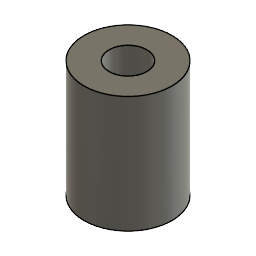
2tslot (Autodesk Fusion 360 archive; units mm, degrees)
design "nggonemotor"
part number: 2026-04-08-22-38-41-699
Autodesk Fusion 360 part; units mm, degrees
cylinder "CylinderPrimitive1" add diameter 18.6 height 24.7 placed x (1, 0, 0) y (0, 0, -1) z (0, 1, 0) at (0, 0, 0)
hole "Hole1" at (0, 24.7, 0) direction (0, -1, 0) diameter 8 depth 10 tip angle 180
hole "Hole2" at (0, 0, 0) direction (0, 1, 0) diameter 4.7 depth 10 tip angle 180
